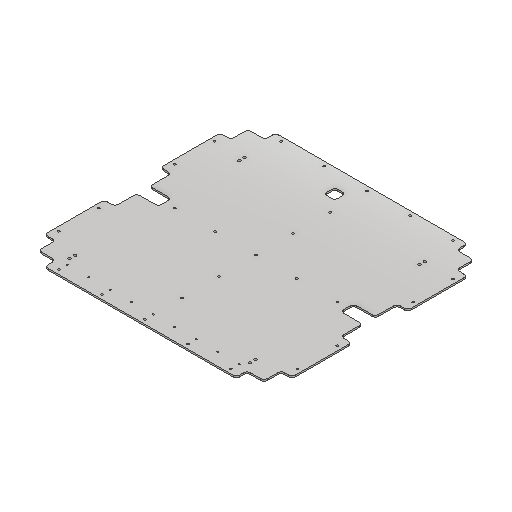
# Autodesk Inventor part: LC_ALU_3mm_Heatbed_Frame_Top_Plate
Saved by Autodesk Inventor 2026.1 (Build 301233000, 233)
## iProperties
Created: 2016-06-21
Part Number: LC_ALU_3mm_Heatbed_Frame_Top_Plate
Material: Ogólny
Document SubType Name: Modeling
Designer: Andrzej
Density: 1 g/cm^3
Appearance: Obrobione - aluminium
Mass: 543.998 g
Surface Area: 3689.65 cm^2
Volume: 543.998 cm^3
Author: Andrzej
Autodesk Inventor part; units mm, degrees
ref_plane "YZ Plane" through (0, 0, 0) normal (1, 0, 0) x (0, 1, 0)
ref_plane "XZ Plane" through (0, 0, 0) normal (0, 1, 0) x (-1, 0, 0)
ref_plane "XY Plane" through (0, 0, 0) normal (0, 0, 1) x (1, 0, 0)
sketch "Szkic1" plane through (0, 0, 0) normal (0, 0, 1) x (1, 0, 0)
  line L0 (-139.3638, 87.0689) -> (-119.3638, 87.0689)
  line L1 (-119.3638, 87.0689) -> (-119.3638, 118.4689)
  line L2 (-119.3638, 118.4689) -> (-87.9638, 118.4689)
  line L3 (-87.9638, 118.4689) -> (-87.9638, 138.4689)
  line L4 (-87.9638, 138.4689) -> (269.2362, 138.4689)
  line L5 (-139.3638, 87.0689) -> (-139.3638, -26.5311)
  line L6 (-139.3638, -26.5311) -> (-119.3638, -26.5311)
  line L7 (-119.3638, -26.5311) -> (-119.3638, -66.5311)
  line L8 (-119.3638, -66.5311) -> (-79.3638, -66.5311)
  line L9 (-79.3638, -66.5311) -> (-79.3638, -86.5311)
  line L10 (-79.3638, -86.5311) -> (-119.3638, -86.5311)
  line L11 (-119.3638, -86.5311) -> (-119.3638, -126.5311)
  line L12 (-119.3638, -126.5311) -> (-139.3638, -126.5311)
  line L13 (-139.3638, -126.5311) -> (-139.3638, -240.1311)
  line L14 (-139.3638, -240.1311) -> (-119.3638, -240.1311)
  line L15 (-119.3638, -240.1311) -> (-119.3638, -271.5311)
  line L16 (-119.3638, -271.5311) -> (-87.9638, -271.5311)
  line L17 (-87.9638, -271.5311) -> (-87.9638, -291.5311)
  line L18 (-87.9638, -291.5311) -> (269.2362, -291.5311)
  line L19 (269.2362, 138.4689) -> (269.2362, 118.4689)
  line L20 (269.2362, 118.4689) -> (300.6362, 118.4689)
  line L21 (300.6362, 118.4689) -> (300.6362, 87.0689)
  line L22 (300.6362, 87.0689) -> (320.6362, 87.0689)
  line L23 (320.6362, 87.0689) -> (320.6362, -26.5311)
  line L24 (269.2362, -291.5311) -> (269.2362, -271.5311)
  line L25 (269.2362, -271.5311) -> (300.6362, -271.5311)
  line L26 (300.6362, -271.5311) -> (300.6362, -240.1311)
  line L27 (300.6362, -240.1311) -> (320.6362, -240.1311)
  line L28 (320.6362, -240.1311) -> (320.6362, -126.5311)
  line L29 (320.6362, -26.5311) -> (300.6362, -26.5311)
  line L30 (300.6362, -26.5311) -> (300.6362, -66.5311)
  line L31 (300.6362, -66.5311) -> (260.6362, -66.5311)
  line L32 (260.6362, -66.5311) -> (260.6362, -86.5311)
  line L33 (260.6362, -86.5311) -> (300.6362, -86.5311)
  line L34 (300.6362, -86.5311) -> (300.6362, -126.5311)
  line L35 (300.6362, -126.5311) -> (320.6362, -126.5311)
  line L36 (267.2362, 136.4689) -> (-85.9638, 136.4689)
  line L37 (-85.9638, 136.4689) -> (-85.9638, 116.4689)
  line L38 (-85.9638, 116.4689) -> (-117.3638, 116.4689)
  line L39 (-117.3638, 116.4689) -> (-117.3638, 85.0689)
  line L40 (-117.3638, 85.0689) -> (-137.3638, 85.0689)
  line L41 (-137.3638, 85.0689) -> (-137.3638, -24.5311)
  line L42 (-137.3638, -24.5311) -> (-117.3638, -24.5311)
  line L43 (-117.3638, -24.5311) -> (-117.3638, -64.5311)
  line L44 (-117.3638, -64.5311) -> (-77.3638, -64.5311)
  line L45 (-77.3638, -64.5311) -> (-77.3638, -88.5311)
  line L46 (-77.3638, -88.5311) -> (-117.3638, -88.5311)
  line L47 (-117.3638, -88.5311) -> (-117.3638, -128.5311)
  line L48 (-117.3638, -128.5311) -> (-137.3638, -128.5311)
  line L49 (-137.3638, -128.5311) -> (-137.3638, -238.1311)
  line L50 (-137.3638, -238.1311) -> (-117.3638, -238.1311)
  line L51 (-117.3638, -238.1311) -> (-117.3638, -269.5311)
  line L52 (-117.3638, -269.5311) -> (-85.9638, -269.5311)
  line L53 (-85.9638, -269.5311) -> (-85.9638, -289.5311)
  line L54 (-85.9638, -289.5311) -> (267.2362, -289.5311)
  line L55 (267.2362, -289.5311) -> (267.2362, -269.5311)
  line L56 (267.2362, -269.5311) -> (298.6362, -269.5311)
  line L57 (298.6362, -269.5311) -> (298.6362, -238.1311)
  line L58 (298.6362, -238.1311) -> (318.6362, -238.1311)
  line L59 (318.6362, -238.1311) -> (318.6362, -128.5311)
  line L60 (318.6362, -128.5311) -> (298.6362, -128.5311)
  line L61 (298.6362, -128.5311) -> (298.6362, -88.5311)
  line L62 (298.6362, -88.5311) -> (258.6362, -88.5311)
  line L63 (258.6362, -88.5311) -> (258.6362, -64.5311)
  line L64 (258.6362, -64.5311) -> (298.6362, -64.5311)
  line L65 (298.6362, -64.5311) -> (298.6362, -24.5311)
  line L66 (298.6362, -24.5311) -> (318.6362, -24.5311)
  line L67 (318.6362, -24.5311) -> (318.6362, 85.0689)
  line L68 (318.6362, 85.0689) -> (298.6362, 85.0689)
  line L69 (298.6362, 85.0689) -> (298.6362, 116.4689)
  line L70 (298.6362, 116.4689) -> (267.2362, 116.4689)
  line L71 (267.2362, 116.4689) -> (267.2362, 136.4689)
  line L72 (60.6362, 103.7689) -> (70.6362, 103.7689)
  line L73 (75.6362, 98.7689) -> (75.6362, 88.7689)
  line L74 (70.6362, 83.7689) -> (60.6362, 83.7689)
  line L75 (55.6362, 88.7689) -> (55.6362, 98.7689)
  arc A0 (60.6362, 103.7689) -> (55.6362, 98.7689) centre (60.6362, 98.7689) ccw
  arc A1 (75.6362, 98.7689) -> (70.6362, 103.7689) centre (70.6362, 98.7689) ccw
  arc A2 (55.6362, 88.7689) -> (60.6362, 83.7689) centre (60.6362, 88.7689) ccw
  arc A3 (70.6362, 83.7689) -> (75.6362, 88.7689) centre (70.6362, 88.7689) ccw
  point P0 (0, 0)
  point P1 (90.6362, 128.4689)
  point P2 (-59.3638, -76.5311)
  point P3 (90.6362, 60.1355)
  point P4 (90.6362, -8.1978)
  point P5 (90.6362, -76.5311)
  point P6 (90.6362, -144.8645)
  point P7 (90.6362, -213.1978)
  point P8 (90.6362, -281.5311)
  point P9 (240.6362, -76.5311)
  point P10 (15.6362, -76.5311)
  point P11 (90.6362, -76.5311)
  point P12 (165.6362, -76.5311)
  point P13 (-75.6638, -243.8311)
  point P14 (-75.6638, 68.7689)
  point P15 (256.9362, 68.7689)
  point P16 (256.9362, -243.8311)
  point P17 (55.6362, 103.7689)
  point P18 (75.6362, 83.7689)
  point P19 (75.6362, 103.7689)
  point P20 (55.6362, 83.7689)
  point P21 (-129.3638, 67.0689)
  point P22 (-129.3638, -6.5311)
  point P23 (-129.3638, -146.5311)
  point P24 (-129.3638, -220.1311)
  point P25 (310.6362, -146.5311)
  point P26 (310.6362, -220.1311)
  point P27 (310.6362, 67.0689)
  point P28 (310.6362, -6.5311)
  point P29 (-67.9638, 128.4689)
  point P30 (11.3362, 128.4689)
  point P31 (169.9362, 128.4689)
  point P32 (249.2362, 128.4689)
  point P33 (-67.9638, -281.5311)
  point P34 (11.3362, -281.5311)
  point P35 (169.9362, -281.5311)
  point P36 (249.2362, -281.5311)
  point P37 (-75.6638, 68.7689)
  point P38 (-75.6638, -253.8311)
  point P39 (256.9362, 58.7689)
  point P40 (256.9362, -253.8311)
  point P41 (-75.6638, 58.7689)
  point P42 (-67.9638, -266.2311)
  point P43 (249.2362, -266.2311)
  point P44 (-28.3138, -266.2311)
  point P45 (11.3362, -266.2311)
  point P46 (50.9862, -266.2311)
  point P47 (90.6362, -266.2311)
  point P48 (130.2862, -266.2311)
  point P49 (169.9362, -266.2311)
  point P50 (209.5862, -266.2311)
  dimension "d0" = 51.4
  dimension "d1" = 51.4
  dimension "d2" = 20
  dimension "d3" = 20
  dimension "d4" = 113.6
  dimension "d5" = 20
  dimension "d6" = 20
  dimension "d7" = 113.6
  dimension "d8" = 20
  dimension "d9" = 40
  dimension "d10" = 40
  dimension "d11" = 40
  dimension "d12" = 20
  dimension "d13" = 20
  dimension "d14" = 51.4
  dimension "d15" = 51.4
  dimension "d16" = 357.2
  dimension "d17" = 357.2
  dimension "d18" = 113.6
  dimension "d19" = 51.4
  dimension "d20" = 51.4
  dimension "d21" = 20
  dimension "d22" = 20
  dimension "d23" = 113.6
  dimension "d24" = 51.4
  dimension "d25" = 51.4
  dimension "d26" = 20
  dimension "d27" = 20
  dimension "d28" = 20
  dimension "d29" = 40
  dimension "d30" = 40
  dimension "d31" = 20
  dimension "d32" = 40
  dimension "d33" = 2
  dimension "d34" = 10
  dimension "d35" = 460
  dimension "d36" = 430
  dimension "d37" = 230
  dimension "d40" = 68.3333
  dimension "d48" = 10
  dimension "d49" = 230
  dimension "d57" = 20
  dimension "d58" = 20
  dimension "d59" = 10
  dimension "d60" = 10
  dimension "d63" = 75
  dimension "d68" = 312.6
  dimension "d69" = 332.6
  dimension "d70" = 312.6
  dimension "d71" = 332.6
  dimension "d72" = 47.7
  dimension "d74" = 47.7
  dimension "d75" = 63.7
  dimension "d76" = 63.7
  dimension "d84" = 20
  dimension "d85" = 20
  dimension "d86" = 15
  dimension "d87" = 15
  dimension "d90" = 5
  dimension "d91" = 5
  dimension "d92" = 5
  dimension "d93" = 5
  dimension "d102" = 10
  dimension "d103" = 10
  constraints: 152 end point, 53 perpendicular, 12 point on line, 8 point on circle, 8 tangent, 7 horizontal, 4 centre point, 4 vertical, 2 parallel, 1 coincident, 50 other
  measures "d0" distance between parallel lines of L4 L0
  measures "d1" distance between parallel lines of L5 L3
  measures "d2" distance between parallel lines of L4 L2
  measures "d3" distance between parallel lines of L5 L1
  measures "d4" distance of L0.start L5.end
  measures "d5" distance of L5.end L6.end
  measures "d6" distance of L8.end L9.end
  measures "d7" distance of L12.end L13.end
  measures "d8" distance of L11.end L12.end
  measures "d9" distance of L6.end L7.end
  measures "d10" distance of L10.end L11.end
  measures "d11" distance between parallel lines of L7 L9
  measures "d12" distance of L13.end L14.end
  measures "d13" distance of L16.end L17.end
  measures "d14" distance between parallel lines of L13 L17
  measures "d15" distance between parallel lines of L18 L14
  measures "d16" distance of L17.end L18.end
  measures "d17" distance of L3.end L4.end
  measures "d18" distance of L22.end L23.end
  measures "d19" distance between parallel lines of L4 L22
  measures "d20" distance from line of L23 L4.end
  measures "d21" distance of L21.end L22.end
  measures "d22" distance of L4.end L19.end
  measures "d23" distance of L27.end L28.end
  measures "d24" distance between parallel lines of L18 L27
  measures "d25" distance between parallel lines of L28 L24
  measures "d26" distance of L18.end L24.end
  measures "d27" distance of L26.end L27.end
  measures "d28" distance of L23.end L29.end
  measures "d29" distance of L29.end L30.end
  measures "d30" distance of L30.end L31.end
  measures "d31" distance of L31.end L32.end
  measures "d32" distance of L33.end L34.end
  measures "d33" distance between parallel lines of L4 L36
  measures "d34" distance from line of L4 point (90.636, 128.469)
  measures "d35" distance between parallel lines of L23 L5
  measures "d36" distance between parallel lines of L18 L4
  measures "d37" distance from line of L5 point (90.636, 128.469)
  measures "d40" distance of point (90.636, 128.469) point (90.636, 60.136)
  measures "d48" distance from line of L18 point (90.636, -281.531)
  measures "d49" distance from line of L13 point (90.636, -281.531)
  measures "d57" distance from line of L9 point (-59.364, -76.531)
  measures "d58" distance from line of point (240.636, -76.531) L32
  measures "d59" distance from line of point (-59.364, -76.531) L8
  measures "d60" distance from line of L31 point (240.636, -76.531)
  measures "d63" distance of point (-59.364, -76.531) point (15.636, -76.531)
  measures "d68" distance of point (-75.664, -243.831) point (-75.664, 68.769)
  measures "d69" distance of point (256.936, -243.831) point (-75.664, -243.831)
  measures "d70" distance of point (256.936, 68.769) point (256.936, -243.831)
  measures "d71" distance of point (256.936, 68.769) point (-75.664, 68.769)
  measures "d72" distance from line of L18 point (-75.664, -243.831)
  measures "d74" distance from line of L18 point (256.936, -243.831)
  measures "d75" distance from line of L13 point (-75.664, -243.831)
  measures "d76" distance from line of L5 point (-75.664, 68.769)
  measures "d84" distance of point (75.636, 83.769) point (55.636, 83.769)
  measures "d85" distance of point (75.636, 103.769) point (75.636, 83.769)
  measures "d86" distance from line of L74 point (-75.664, 68.769)
  measures "d87" distance from line of point (90.636, 60.136) L73
  measures "d90" radius of A0
  measures "d91" radius of A1
  measures "d92" radius of A2
  measures "d93" radius of A3
  measures "d102" distance from line of L4 point (169.936, 128.469)
  measures "d103" distance from line of L4 point (249.236, 128.469)
extrude "Wyciągnięcie proste1" add sketch "Szkic1" along normal blind 3 contours L71 L70 L69 L68 L67 L66 L65 L64 L63 L62 L61 L60 L59 L58 L57 L56 L55 L54 L53 L52 L51 L50 L49 L48 L47 L46 L45 L44 L43 L42 L41 L40 L39 L38 L37 L36 | L72 A1 L73 A3 L74 A2 L75 A0
fillet "Zaokrąglenie1" radius 6 36 edges at (267.2362, -289.5311, 1.5) (267.2362, -269.5311, 1.5) (298.6362, -269.5311, 1.5) (298.6362, -238.1311, 1.5) (318.6362, -238.1311, 1.5) (318.6362, -128.5311, 1.5) (298.6362, -128.5311, 1.5) (298.6362, -88.5311, 1.5) (258.6362, -88.5311, 1.5) (258.6362, -64.5311, 1.5) (298.6362, -64.5311, 1.5) (298.6362, -24.5311, 1.5) (318.6362, -24.5311, 1.5) (318.6362, 85.0689, 1.5) (298.6362, 85.0689, 1.5) (298.6362, 116.4689, 1.5) (267.2362, 116.4689, 1.5) (267.2362, 136.4689, 1.5) (-85.9638, 136.4689, 1.5) (-85.9638, 116.4689, 1.5) (-117.3638, 116.4689, 1.5) (-117.3638, 85.0689, 1.5) (-137.3638, 85.0689, 1.5) (-137.3638, -24.5311, 1.5) (-117.3638, -24.5311, 1.5) (-117.3638, -64.5311, 1.5) (-77.3638, -64.5311, 1.5) (-77.3638, -88.5311, 1.5) (-117.3638, -88.5311, 1.5) (-117.3638, -128.5311, 1.5) (-137.3638, -128.5311, 1.5) (-137.3638, -238.1311, 1.5) (-117.3638, -238.1311, 1.5) (-117.3638, -269.5311, 1.5) (-85.9638, -269.5311, 1.5) (-85.9638, -289.5311, 1.5)
hole "Otwór1" at (90.6362, 128.4689, 0) at (-59.3638, -76.5311, 0) at (90.6362, 60.1355, 0) at (90.6362, -8.1978, 0) at (90.6362, -76.5311, 0) at (90.6362, -144.8645, 0) at (90.6362, -213.1978, 0) at (90.6362, -281.5311, 0) at (15.6362, -76.5311, 0) at (240.6362, -76.5311, 0) at (165.6362, -76.5311, 0) at (249.2362, 128.4689, 0) at (169.9362, 128.4689, 0) at (11.3362, 128.4689, 0) at (-67.9638, 128.4689, 0) at (-129.3638, 67.0689, 0) at (-129.3638, -6.5311, 0) at (-129.3638, -146.5311, 0) at (-129.3638, -220.1311, 0) at (-67.9638, -281.5311, 0) at (11.3362, -281.5311, 0) at (169.9362, -281.5311, 0) at (249.2362, -281.5311, 0) at (310.6362, -220.1311, 0) at (310.6362, -146.5311, 0) at (310.6362, -6.5311, 0) at (310.6362, 67.0689, 0) direction (0, 0, 1) diameter 4 end through all
extrude "Wyciągnięcie proste2" cut sketch "Szkic1" along normal blind 10 contours L72 A1 L73 A3 L74 A2 L75 A0
hole "Otwór3" at (256.9362, -243.8311, 0) at (256.9362, 68.7689, 0) at (-75.6638, 68.7689, 0) at (-75.6638, -243.8311, 0) at (-75.6638, -253.8311, 0) at (256.9362, -253.8311, 0) at (256.9362, 58.7689, 0) at (-75.6638, 58.7689, 0) direction (0, 0, 1) diameter 5 end through all
hole "Otwór4" at (-67.9638, -266.2311, 0) at (-28.3138, -266.2311, 0) at (50.9862, -266.2311, 0) at (11.3362, -266.2311, 0) at (130.2862, -266.2311, 0) at (90.6362, -266.2311, 0) at (209.5862, -266.2311, 0) at (169.9362, -266.2311, 0) at (249.2362, -266.2311, 0) direction (0, 0, 1) diameter 3 end through all
equation "\"d1\" = d0"
equation "\"d7\" = d4"
equation "\"d10\" = d9"
equation "\"d13\" = d12"
equation "\"d14\" = d0"
equation "\"d15\" = d14"
equation "\"d17\" = d16"
equation "\"d18\" = d4"
equation "\"d19\" = d0"
equation "\"d20\" = d0"
equation "\"d21\" = d2"
equation "\"d23\" = d4"
equation "\"d24\" = d0"
equation "\"d25\" = d0"
equation "\"d26\" = d2"
equation "\"d27\" = d26"
equation "\"d37\" = 0.5 * d35"
equation "\"d49\" = d37"
equation "\"d70\" = d68"
equation "\"d71\" = d69"
equation "\"d74\" = d72"
equation "\"d76\" = d75"
